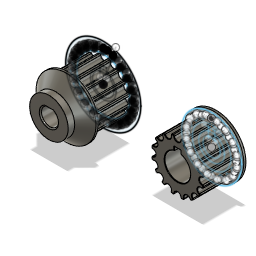
htd5m (Autodesk Fusion 360 design; units mm, degrees)
Autodesk Fusion 360 part; units mm, degrees
sketch "Sketch1" plane through (0, 0, 0) normal (0, 0, 1) x (1, 0, 0)
  circle A0 centre (0, 0) radius 15.345 construction
  circle A1 centre (0, 0) radius 13.285 construction
  line L0 (0, 0) -> (0, 15.345) construction
  circle A2 centre (0, 14.81) radius 1.525 construction
  line L1 (0, 0) -> (5.8121, 17.8879)
  circle A3 centre (4.5765, 14.0851) radius 1.525 construction
  circle A4 centre (2.7586, 14.6956) radius 0.3927 construction
  circle A5 centre (1.9549, 14.7863) radius 0.43 construction
  arc A6 (0, 13.285) -> (1.5249, 14.7915) centre (0, 14.81) ccw
  arc A7 (2.0112, 15.2126) -> (1.5249, 14.7915) centre (1.9549, 14.7863) ccw
  arc A8 (3.1309, 14.5706) -> (2.8311, 15.0816) centre (2.7586, 14.6956) ccw
  arc A9 (3.1309, 14.5706) -> (4.1053, 12.6348) centre (4.5765, 14.0851) ccw
  line L2 (2.8311, 15.0816) -> (2.0112, 15.2126)
  arc A10 (-1.5249, 14.825) -> (0, 13.285) centre (0, 14.81) ccw
  arc A11 (-1.5249, 14.825) -> (-1.968, 15.2183) centre (-1.9176, 14.8288) ccw
  line L3 (-1.968, 15.2183) -> (-2.7882, 15.0896)
  arc A12 (-2.7882, 15.0896) -> (-3.1206, 14.5388) centre (-2.7101, 14.6667) ccw
  arc A13 (-4.1053, 12.6348) -> (-3.1206, 14.5388) centre (-4.5765, 14.0851) ccw
  arc A14 (-6.0315, 13.6282) -> (-4.1053, 12.6348) centre (-4.5765, 14.0851) ccw
  arc A15 (-6.0315, 13.6282) -> (-6.5743, 13.8653) centre (-6.4061, 13.5105) ccw
  line L4 (-6.5743, 13.8653) -> (-7.3147, 13.4894)
  arc A16 (-7.3147, 13.4894) -> (-7.4606, 12.8629) centre (-7.1097, 13.1114) ccw
  arc A17 (-7.8087, 10.7478) -> (-7.4606, 12.8629) centre (-8.7051, 11.9815) ccw
  arc A18 (-9.9476, 11.0973) -> (-7.8087, 10.7478) centre (-8.7051, 11.9815) ccw
  arc A19 (-9.9476, 11.0973) -> (-10.5372, 11.1551) centre (-10.2675, 10.8697) ccw
  line L5 (-10.5372, 11.1551) -> (-11.1251, 10.5689)
  arc A20 (-11.1251, 10.5689) -> (-11.0703, 9.9279) centre (-10.8134, 10.2727) ccw
  arc A21 (-10.7478, 7.8087) -> (-11.0703, 9.9279) centre (-11.9815, 8.7051) ccw
  arc A22 (-12.89, 7.4802) -> (-10.7478, 7.8087) centre (-11.9815, 8.7051) ccw
  arc A23 (-12.89, 7.4802) -> (-13.4686, 7.353) centre (-13.1239, 7.1648) ccw
  line L6 (-13.4686, 7.353) -> (-13.8466, 6.6137)
  arc A24 (-13.8466, 6.6137) -> (-13.5964, 6.0211) centre (-13.4586, 6.4284) ccw
  arc A25 (-12.6348, 4.1053) -> (-13.5964, 6.0211) centre (-14.0851, 4.5765) ccw
  arc A26 (-14.5706, 3.1309) -> (-12.6348, 4.1053) centre (-14.0851, 4.5765) ccw
  arc A27 (-14.5706, 3.1309) -> (-15.0816, 2.8311) centre (-14.6956, 2.7586) ccw
  line L7 (-15.0816, 2.8311) -> (-15.2126, 2.0112)
  arc A28 (-15.2126, 2.0112) -> (-14.7915, 1.5249) centre (-14.7863, 1.9549) ccw
  arc A29 (-13.285, 0) -> (-14.7915, 1.5249) centre (-14.81, 0) ccw
  arc A30 (-14.825, -1.5249) -> (-13.285, 0) centre (-14.81, 0) ccw
  arc A31 (-14.825, -1.5249) -> (-15.2183, -1.968) centre (-14.8288, -1.9176) ccw
  line L8 (-15.2183, -1.968) -> (-15.0896, -2.7882)
  arc A32 (-15.0896, -2.7882) -> (-14.5388, -3.1206) centre (-14.6667, -2.7101) ccw
  arc A33 (-12.6348, -4.1053) -> (-14.5388, -3.1206) centre (-14.0851, -4.5765) ccw
  arc A34 (-13.6282, -6.0315) -> (-12.6348, -4.1053) centre (-14.0851, -4.5765) ccw
  arc A35 (-13.6282, -6.0315) -> (-13.8653, -6.5743) centre (-13.5105, -6.4061) ccw
  line L9 (-13.8653, -6.5743) -> (-13.4894, -7.3147)
  arc A36 (-13.4894, -7.3147) -> (-12.8629, -7.4606) centre (-13.1114, -7.1097) ccw
  arc A37 (-10.7478, -7.8087) -> (-12.8629, -7.4606) centre (-11.9815, -8.7051) ccw
  arc A38 (-11.0973, -9.9476) -> (-10.7478, -7.8087) centre (-11.9815, -8.7051) ccw
  arc A39 (-11.0973, -9.9476) -> (-11.1551, -10.5372) centre (-10.8697, -10.2675) ccw
  line L10 (-11.1551, -10.5372) -> (-10.5689, -11.1251)
  arc A40 (-10.5689, -11.1251) -> (-9.9279, -11.0703) centre (-10.2727, -10.8134) ccw
  arc A41 (-7.8087, -10.7478) -> (-9.9279, -11.0703) centre (-8.7051, -11.9815) ccw
  arc A42 (-7.4802, -12.89) -> (-7.8087, -10.7478) centre (-8.7051, -11.9815) ccw
  arc A43 (-7.4802, -12.89) -> (-7.353, -13.4686) centre (-7.1648, -13.1239) ccw
  line L11 (-7.353, -13.4686) -> (-6.6137, -13.8466)
  arc A44 (-6.6137, -13.8466) -> (-6.0211, -13.5964) centre (-6.4284, -13.4586) ccw
  arc A45 (-4.1053, -12.6348) -> (-6.0211, -13.5964) centre (-4.5765, -14.0851) ccw
  arc A46 (-3.1309, -14.5706) -> (-4.1053, -12.6348) centre (-4.5765, -14.0851) ccw
  arc A47 (-3.1309, -14.5706) -> (-2.8311, -15.0816) centre (-2.7586, -14.6956) ccw
  line L12 (-2.8311, -15.0816) -> (-2.0112, -15.2126)
  arc A48 (-2.0112, -15.2126) -> (-1.5249, -14.7915) centre (-1.9549, -14.7863) ccw
  arc A49 (0, -13.285) -> (-1.5249, -14.7915) centre (0, -14.81) ccw
  arc A50 (1.5249, -14.825) -> (0, -13.285) centre (0, -14.81) ccw
  arc A51 (1.5249, -14.825) -> (1.968, -15.2183) centre (1.9176, -14.8288) ccw
  line L13 (1.968, -15.2183) -> (2.7882, -15.0896)
  arc A52 (2.7882, -15.0896) -> (3.1206, -14.5388) centre (2.7101, -14.6667) ccw
  arc A53 (4.1053, -12.6348) -> (3.1206, -14.5388) centre (4.5765, -14.0851) ccw
  arc A54 (6.0315, -13.6282) -> (4.1053, -12.6348) centre (4.5765, -14.0851) ccw
  arc A55 (6.0315, -13.6282) -> (6.5743, -13.8653) centre (6.4061, -13.5105) ccw
  line L14 (6.5743, -13.8653) -> (7.3147, -13.4894)
  arc A56 (7.3147, -13.4894) -> (7.4606, -12.8629) centre (7.1097, -13.1114) ccw
  arc A57 (7.8087, -10.7478) -> (7.4606, -12.8629) centre (8.7051, -11.9815) ccw
  arc A58 (9.9476, -11.0973) -> (7.8087, -10.7478) centre (8.7051, -11.9815) ccw
  arc A59 (9.9476, -11.0973) -> (10.5372, -11.1551) centre (10.2675, -10.8697) ccw
  line L15 (10.5372, -11.1551) -> (11.1251, -10.5689)
  arc A60 (11.1251, -10.5689) -> (11.0703, -9.9279) centre (10.8134, -10.2727) ccw
  arc A61 (10.7478, -7.8087) -> (11.0703, -9.9279) centre (11.9815, -8.7051) ccw
  arc A62 (12.89, -7.4802) -> (10.7478, -7.8087) centre (11.9815, -8.7051) ccw
  arc A63 (12.89, -7.4802) -> (13.4686, -7.353) centre (13.1239, -7.1648) ccw
  line L16 (13.4686, -7.353) -> (13.8466, -6.6137)
  arc A64 (13.8466, -6.6137) -> (13.5964, -6.0211) centre (13.4586, -6.4284) ccw
  arc A65 (12.6348, -4.1053) -> (13.5964, -6.0211) centre (14.0851, -4.5765) ccw
  arc A66 (14.5706, -3.1309) -> (12.6348, -4.1053) centre (14.0851, -4.5765) ccw
  arc A67 (14.5706, -3.1309) -> (15.0816, -2.8311) centre (14.6956, -2.7586) ccw
  line L17 (15.0816, -2.8311) -> (15.2126, -2.0112)
  arc A68 (15.2126, -2.0112) -> (14.7915, -1.5249) centre (14.7863, -1.9549) ccw
  arc A69 (13.285, 0) -> (14.7915, -1.5249) centre (14.81, 0) ccw
  arc A70 (14.825, 1.5249) -> (13.285, 0) centre (14.81, 0) ccw
  arc A71 (14.825, 1.5249) -> (15.2183, 1.968) centre (14.8288, 1.9176) ccw
  line L18 (15.2183, 1.968) -> (15.0896, 2.7882)
  arc A72 (15.0896, 2.7882) -> (14.5388, 3.1206) centre (14.6667, 2.7101) ccw
  arc A73 (12.6348, 4.1053) -> (14.5388, 3.1206) centre (14.0851, 4.5765) ccw
  arc A74 (13.6282, 6.0315) -> (12.6348, 4.1053) centre (14.0851, 4.5765) ccw
  arc A75 (13.6282, 6.0315) -> (13.8653, 6.5743) centre (13.5105, 6.4061) ccw
  line L19 (13.8653, 6.5743) -> (13.4894, 7.3147)
  arc A76 (13.4894, 7.3147) -> (12.8629, 7.4606) centre (13.1114, 7.1097) ccw
  arc A77 (10.7478, 7.8087) -> (12.8629, 7.4606) centre (11.9815, 8.7051) ccw
  arc A78 (11.0973, 9.9476) -> (10.7478, 7.8087) centre (11.9815, 8.7051) ccw
  arc A79 (11.0973, 9.9476) -> (11.1551, 10.5372) centre (10.8697, 10.2675) ccw
  line L20 (11.1551, 10.5372) -> (10.5689, 11.1251)
  arc A80 (10.5689, 11.1251) -> (9.9279, 11.0703) centre (10.2727, 10.8134) ccw
  arc A81 (7.8087, 10.7478) -> (9.9279, 11.0703) centre (8.7051, 11.9815) ccw
  arc A82 (7.4802, 12.89) -> (7.8087, 10.7478) centre (8.7051, 11.9815) ccw
  arc A83 (7.4802, 12.89) -> (7.353, 13.4686) centre (7.1648, 13.1239) ccw
  line L21 (7.353, 13.4686) -> (6.6137, 13.8466)
  arc A84 (6.6137, 13.8466) -> (6.0211, 13.5964) centre (6.4284, 13.4586) ccw
  arc A85 (4.1053, 12.6348) -> (6.0211, 13.5964) centre (4.5765, 14.0851) ccw
  circle A86 centre (0, 0) radius 17.5
  circle A87 centre (0, 0) radius 5
  line L22 (2.1794, 4.5) -> (-2.1794, 4.5)
  circle A88 centre (0, 0) radius 6
  line L23 (-1.5, 7.48) -> (1.5, 7.48)
  line L24 (-1.5, 7.48) -> (-1.5, 2.3316)
  line L25 (1.5, 7.48) -> (1.5, 3.2749)
  circle A89 centre (0, 0) radius 12.3184
  circle A90 centre (50.6261, -0.0294) radius 10.15 construction
  line L26 (50.6261, -0.0294) -> (50.6261, 12.1806) construction
  arc A91 (48.6006, 12.0114) -> (49.1018, 11.6002) centre (48.672, 11.5873) ccw construction
  arc A92 (49.1018, 11.6002) -> (48.6006, 12.0114) centre (48.672, 11.5873) ccw
  arc A93 (49.1683, 12.0932) -> (48.6006, 12.0114) centre (50.6261, -0.0294) ccw
  arc A94 (52.6516, 12.0114) -> (52.1504, 11.6002) centre (52.5802, 11.5873) ccw
  arc A95 (52.1504, 11.6002) -> (52.6516, 12.0114) centre (52.5802, 11.5873) ccw construction
  arc A96 (48.6006, 12.0114) -> (52.6516, 12.0114) centre (50.6261, -0.0294) ccw
  arc A97 (52.0839, 12.0932) -> (49.1683, 12.0932) centre (50.6261, -0.0294) ccw
  arc A98 (52.6516, 12.0114) -> (52.0839, 12.0932) centre (50.6261, -0.0294) ccw
  arc A99 (52.0839, 12.0932) -> (49.1683, 12.0932) centre (50.6261, 11.6456) ccw construction
  arc A100 (49.1683, 12.0932) -> (49.1018, 11.6002) centre (50.6261, 11.6456) ccw
  arc A101 (52.1504, 11.6002) -> (52.0839, 12.0932) centre (50.6261, 11.6456) ccw
  arc A102 (50.6261, 10.1206) -> (52.1504, 11.6002) centre (50.6261, 11.6456) ccw
  arc A103 (49.1018, 11.6002) -> (50.6261, 10.1206) centre (50.6261, 11.6456) ccw
  arc A104 (44.7674, 10.1316) -> (46.7419, 9.3479) centre (46.1583, 10.7569) ccw
  arc A105 (46.7419, 9.3479) -> (47.5839, 11.2982) centre (46.1583, 10.7569) ccw
  arc A106 (47.8896, 11.8699) -> (47.5839, 11.2982) centre (47.9859, 11.4509) ccw
  arc A107 (44.7674, 10.1316) -> (44.147, 10.3197) centre (44.3752, 9.9553) ccw
  arc A108 (41.3249, 7.1161) -> (43.449, 7.1477) centre (42.3706, 8.226) ccw
  arc A109 (43.449, 7.1477) -> (43.4806, 9.2718) centre (42.3706, 8.226) ccw
  arc A110 (43.5442, 9.9169) -> (43.4806, 9.2718) centre (43.7936, 9.5667) ccw
  arc A111 (41.3249, 7.1161) -> (40.6797, 7.0525) centre (41.03, 6.8031) ccw
  arc A112 (39.2984, 3.0127) -> (41.2487, 3.8548) centre (39.8398, 4.4384) ccw
  arc A113 (41.2487, 3.8548) -> (40.4651, 5.8293) centre (39.8398, 4.4384) ccw
  arc A114 (40.2769, 6.4497) -> (40.4651, 5.8293) centre (40.6414, 6.2215) ccw
  arc A115 (39.2984, 3.0127) -> (38.7267, 2.7071) centre (39.1458, 2.6107) ccw
  arc A116 (38.9965, -1.5538) -> (40.4761, -0.0294) centre (38.9511, -0.0294) ccw
  arc A117 (40.4761, -0.0294) -> (38.9965, 1.4949) centre (38.9511, -0.0294) ccw
  arc A118 (38.5853, 1.996) -> (38.9965, 1.4949) centre (39.0093, 1.9247) ccw
  arc A119 (38.9965, -1.5538) -> (38.5853, -2.0549) centre (39.0093, -1.9836) ccw
  arc A120 (40.4651, -5.8882) -> (41.2487, -3.9137) centre (39.8398, -4.4973) ccw
  arc A121 (41.2487, -3.9137) -> (39.2984, -3.0716) centre (39.8398, -4.4973) ccw
  arc A122 (38.7267, -2.766) -> (39.2984, -3.0716) centre (39.1458, -2.6696) ccw
  arc A123 (40.4651, -5.8882) -> (40.2769, -6.5085) centre (40.6414, -6.2804) ccw
  arc A124 (43.4806, -9.3307) -> (43.449, -7.2066) centre (42.3706, -8.2849) ccw
  arc A125 (43.449, -7.2066) -> (41.3249, -7.1749) centre (42.3706, -8.2849) ccw
  arc A126 (40.6797, -7.1114) -> (41.3249, -7.1749) centre (41.03, -6.862) ccw
  arc A127 (43.4806, -9.3307) -> (43.5442, -9.9758) centre (43.7936, -9.6255) ccw
  arc A128 (47.5839, -11.3571) -> (46.7419, -9.4068) centre (46.1583, -10.8157) ccw
  arc A129 (46.7419, -9.4068) -> (44.7674, -10.1904) centre (46.1583, -10.8157) ccw
  arc A130 (44.147, -10.3786) -> (44.7674, -10.1904) centre (44.3752, -10.0141) ccw
  arc A131 (47.5839, -11.3571) -> (47.8896, -11.9288) centre (47.9859, -11.5098) ccw
  arc A132 (52.1504, -11.659) -> (50.6261, -10.1794) centre (50.6261, -11.7044) ccw
  arc A133 (50.6261, -10.1794) -> (49.1018, -11.659) centre (50.6261, -11.7044) ccw
  arc A134 (48.6006, -12.0703) -> (49.1018, -11.659) centre (48.672, -11.6462) ccw
  arc A135 (52.1504, -11.659) -> (52.6516, -12.0703) centre (52.5802, -11.6462) ccw
  arc A136 (56.4849, -10.1904) -> (54.5103, -9.4068) centre (55.0939, -10.8157) ccw
  arc A137 (54.5103, -9.4068) -> (53.6683, -11.3571) centre (55.0939, -10.8157) ccw
  arc A138 (53.3627, -11.9288) -> (53.6683, -11.3571) centre (53.2663, -11.5098) ccw
  arc A139 (56.4849, -10.1904) -> (57.1052, -10.3786) centre (56.877, -10.0141) ccw
  arc A140 (59.9273, -7.1749) -> (57.8032, -7.2066) centre (58.8816, -8.2849) ccw
  arc A141 (57.8032, -7.2066) -> (57.7716, -9.3307) centre (58.8816, -8.2849) ccw
  arc A142 (57.708, -9.9758) -> (57.7716, -9.3307) centre (57.4586, -9.6255) ccw
  arc A143 (59.9273, -7.1749) -> (60.5725, -7.1114) centre (60.2222, -6.862) ccw
  arc A144 (61.9538, -3.0716) -> (60.0035, -3.9137) centre (61.4124, -4.4973) ccw
  arc A145 (60.0035, -3.9137) -> (60.7871, -5.8882) centre (61.4124, -4.4973) ccw
  arc A146 (60.9753, -6.5085) -> (60.7871, -5.8882) centre (60.6108, -6.2804) ccw
  arc A147 (61.9538, -3.0716) -> (62.5255, -2.766) centre (62.1064, -2.6696) ccw
  arc A148 (62.2557, 1.4949) -> (60.7761, -0.0294) centre (62.3011, -0.0294) ccw
  arc A149 (60.7761, -0.0294) -> (62.2557, -1.5538) centre (62.3011, -0.0294) ccw
  arc A150 (62.6669, -2.0549) -> (62.2557, -1.5538) centre (62.2429, -1.9836) ccw
  arc A151 (62.2557, 1.4949) -> (62.6669, 1.996) centre (62.2429, 1.9247) ccw
  arc A152 (60.7871, 5.8293) -> (60.0035, 3.8548) centre (61.4124, 4.4384) ccw
  arc A153 (60.0035, 3.8548) -> (61.9538, 3.0127) centre (61.4124, 4.4384) ccw
  arc A154 (62.5255, 2.7071) -> (61.9538, 3.0127) centre (62.1064, 2.6107) ccw
  arc A155 (60.7871, 5.8293) -> (60.9753, 6.4497) centre (60.6108, 6.2215) ccw
  arc A156 (57.7716, 9.2718) -> (57.8032, 7.1477) centre (58.8816, 8.226) ccw
  arc A157 (57.8032, 7.1477) -> (59.9273, 7.1161) centre (58.8816, 8.226) ccw
  arc A158 (60.5725, 7.0525) -> (59.9273, 7.1161) centre (60.2222, 6.8031) ccw
  arc A159 (57.7716, 9.2718) -> (57.708, 9.9169) centre (57.4586, 9.5667) ccw
  arc A160 (53.6683, 11.2982) -> (54.5103, 9.3479) centre (55.0939, 10.7569) ccw
  arc A161 (54.5103, 9.3479) -> (56.4849, 10.1316) centre (55.0939, 10.7569) ccw
  arc A162 (57.1052, 10.3197) -> (56.4849, 10.1316) centre (56.877, 9.9553) ccw
  arc A163 (53.6683, 11.2982) -> (53.3627, 11.8699) centre (53.2663, 11.4509) ccw
  circle A164 centre (50.6261, -0.0294) radius 4
  circle A165 centre (50.6261, -0.0294) radius 6
  line L27 (48.6896, 3.4706) -> (52.5626, 3.4706)
  line L28 (47.069, 7.4506) -> (54.0561, 7.4506)
  line L29 (49.1261, 7.4506) -> (49.1261, 2.8308)
  line L30 (52.1261, 7.4506) -> (52.1261, 2.9509)
  circle A166 centre (50.6261, -0.0294) radius 14
  circle A167 centre (50.6261, -0.0294) radius 9
  dimension "d1" = 30.69
  dimension "d3" = 3.05
  dimension "d6" = 26.57
  dimension "d7" = 18
  dimension "d8" = 3.05
  dimension "d9" = 0.86
  dimension "d11" = 360
  dimension "d14" = 35
  dimension "d17" = 10
  dimension "d18" = 4.5
  dimension "d22" = 12
  dimension "d23" = 1.5
  dimension "d24" = 1.5
  dimension "d25" = 7.48
  dimension "d44" = 24.42
  dimension "d45" = 20.3
  dimension "d46" = 3.05
  dimension "d47" = 0.86
  dimension "d48" = 0.86
  dimension "d50" = 360
  dimension "d51" = 8
  dimension "d52" = 12
  dimension "d53" = 3.5
  dimension "d54" = 7.48
  dimension "d55" = 1.5
  dimension "d56" = 1.5
  dimension "d57" = 28
  dimension "d74" = 18
  constraint coincident A0.centre A1.centre
  constraint coincident A0 L0.end
  constraint vertical L0
  constraint coincident L0 A2.centre
  constraint tangent A1 A2
  constraint coincident L1 A3.centre
  constraint tangent A1 A3
  constraint tangent A3 A4
  constraint tangent A0 A4
  constraint tangent A0 A5
  constraint tangent A2 A5
  constraint coincident A2 A6.end
  constraint coincident A5 A6.end
  constraint coincident A1 A6.start
  constraint coincident L0 A6.start
  constraint coincident A5.centre A7.centre
  constraint coincident A0 A8.end
  constraint coincident A4 A8.end
  constraint coincident A4.centre A8.centre
  constraint coincident A3 A9.end
  constraint coincident A1 A9.end
  constraint coincident L1 A9.end
  constraint coincident A3.centre A9.centre
  constraint concentric A0 A86
  constraint concentric A86 A87
  constraint coincident A87 L22.start
  constraint coincident A87 L22.end
  constraint horizontal L22
  constraint concentric A86 A88
  constraint perpendicular L0 L23
  constraint perpendicular L23 L24
  constraint perpendicular L23 L25
  constraint concentric A86 A89
  constraint concentric A90 A96
  constraint coincident A90.centre L26.start
  constraint coincident L26.end A96
  constraint vertical L26
  constraint coincident L26 A99.centre
  constraint tangent A90 A100
  constraint tangent A94 A96
  constraint tangent A94 A100
  constraint tangent A91 A96
  constraint tangent A91 A100
  constraint concentric A91 A92
  constraint concentric A93 A96
  constraint coincident A94.end A100
  constraint concentric A94 A95
  constraint concentric A96 A97
  constraint concentric A96 A98
  constraint concentric A99 A100
  constraint coincident A90 A102.start
  constraint concentric A100 A101
  constraint concentric A100 A102
  constraint concentric A100 A103
  constraint concentric A98 A164
  constraint concentric A98 A165
  constraint coincident A164 L27.start
  constraint coincident A164 L27.end
  constraint horizontal L27
  constraint perpendicular L26 L28
  constraint coincident L28 L29.start
  constraint perpendicular L28 L29
  constraint coincident L28 L30.start
  constraint perpendicular L28 L30
  constraint concentric A165 A166
  constraint concentric A90 A167
  measures "d1" diameter of A0
  measures "d3" diameter of A2
  measures "d6" diameter of A1
  measures "d7" angle of L0 L1
  measures "d8" diameter of A3
  measures "d9" diameter of A5
  measures "d14" diameter of A86
  measures "d17" diameter of A87
  measures "d18" distance of A0.centre L22
  measures "d22" diameter of A88
  measures "d23" distance of L0 L24
  measures "d24" distance of L0 L25
  measures "d25" distance of A0.centre L23
  measures "d44" diameter of A96
  measures "d45" diameter of A90
  measures "d46" diameter of A100
  measures "d47" diameter of A94
  measures "d48" diameter of A91
  measures "d51" diameter of A164
  measures "d52" diameter of A165
  measures "d53" distance of A90.centre L27
  measures "d54" distance of A90.centre L28
  measures "d55" distance of L26 L30
  measures "d56" distance of L26 L29
  measures "d57" diameter of A166
  measures "d74" diameter of A167
extrude "Extrude7" add sketch "Sketch1" along normal blind 16 contours A92 A94 A96 A102 A103 A104 A105 A106 A107 A108 A109 A110 A111 A112 A113 A114 A115 A116 A117 A118 A119 A120 A121 A122 A123 A124 A125 A126 A127 A128 A129 A130 A131 A132 A133 A134 A135 A136 A137 A138 A139 A140 A141 A142 A143 A144 A145 A146 A147 A148 A149 A150 A151 A152 A153 A154 A155 A156 A157 A158 A159 A160 A161 A162 A163 | A167 makes body 1
extrude "Extrude2" add sketch "Sketch1" against normal blind 2 separate body contours L1 A87 L22 L24 L25 | L1 L22 L25 | A87 L22 | L1 A87 L25 | L1 A87 L22 L25 | A87 L22 L24 | L1 A87 A88 L25 | L1 A87 A88 L24 | A87 A88 L24 L25 | A88 L23 L24 L25 | A6 A7 A8 A9 L2 A10 A11 L3 A12 A13 A14 A15 L4 A16 A17 A18 A19 L5 A20 A21 A22 A23 L6 A24 A25 A26 A27 L7 A28 A29 A30 A31 L8 A32 A33 A34 A35 L9 A36 A37 A38 A39 L10 A40 A41 A42 A43 L11 A44 A45 A46 A47 L12 A48 A49 A50 A51 L13 A52 A53 A54 A55 L14 A56 A57 A58 A59 L15 A60 A61 A62 A63 L16 A64 A65 A66 A67 L17 A68 A69 A70 A71 L18 A72 A73 A74 A75 L19 A76 A77 A78 A79 L20 A80 A81 A82 A83 L21 A84 A85 | A86 | A89 makes body 2
extrude "Extrude1" add sketch "Sketch1" along normal blind 16 separate body contours L1 A87 L22 L24 L25 | L1 L22 L25 | A87 L22 | L1 A87 L25 | L1 A87 L22 L25 | A87 L22 L24 | L1 A87 A88 L25 | L1 A87 A88 L24 | A87 A88 L24 L25 | A88 L23 L24 L25 | A6 A7 A8 A9 L2 A10 A11 L3 A12 A13 A14 A15 L4 A16 A17 A18 A19 L5 A20 A21 A22 A23 L6 A24 A25 A26 A27 L7 A28 A29 A30 A31 L8 A32 A33 A34 A35 L9 A36 A37 A38 A39 L10 A40 A41 A42 A43 L11 A44 A45 A46 A47 L12 A48 A49 A50 A51 L13 A52 A53 A54 A55 L14 A56 A57 A58 A59 L15 A60 A61 A62 A63 L16 A64 A65 A66 A67 L17 A68 A69 A70 A71 L18 A72 A73 A74 A75 L19 A76 A77 A78 A79 L20 A80 A81 A82 A83 L21 A84 A85 | A89 makes body 3
extrude "Extrude3" cut sketch "Sketch1" along normal blind 120 from surface at -2 contours A87 L22 bodies 2 3
combine "Combine1" operation add target body 3 tool bodies 2
extrude "Extrude4" add sketch "Sketch1" along normal blind 16 from surface at 80 separate body contours A6 A7 A8 A9 L2 A10 A11 L3 A12 A13 A14 A15 L4 A16 A17 A18 A19 L5 A20 A21 A22 A23 L6 A24 A25 A26 A27 L7 A28 A29 A30 A31 L8 A32 A33 A34 A35 L9 A36 A37 A38 A39 L10 A40 A41 A42 A43 L11 A44 A45 A46 A47 L12 A48 A49 A50 A51 L13 A52 A53 A54 A55 L14 A56 A57 A58 A59 L15 A60 A61 A62 A63 L16 A64 A65 A66 A67 L17 A68 A69 A70 A71 L18 A72 A73 A74 A75 L19 A76 A77 A78 A79 L20 A80 A81 A82 A83 L21 A84 A85 | A89 makes body 4
extrude "Extrude5" add sketch "Sketch1" against normal blind 2 from surface at 80 contours A6 A7 A8 A9 L2 A10 A11 L3 A12 A13 A14 A15 L4 A16 A17 A18 A19 L5 A20 A21 A22 A23 L6 A24 A25 A26 A27 L7 A28 A29 A30 A31 L8 A32 A33 A34 A35 L9 A36 A37 A38 A39 L10 A40 A41 A42 A43 L11 A44 A45 A46 A47 L12 A48 A49 A50 A51 L13 A52 A53 A54 A55 L14 A56 A57 A58 A59 L15 A60 A61 A62 A63 L16 A64 A65 A66 A67 L17 A68 A69 A70 A71 L18 A72 A73 A74 A75 L19 A76 A77 A78 A79 L20 A80 A81 A82 A83 L21 A84 A85 | A86 | A89 bodies 4
extrude "Extrude6" add sketch "Sketch1" against normal blind 8 from surface at -2 contours L1 A87 L22 L24 L25 | L1 L22 L25 | L1 A87 L25 | L1 A87 L22 L25 | A87 L22 L24 | L1 A87 A88 L25 | L1 A87 A88 L24 | A87 A88 L24 L25 | A88 L23 L24 L25 | A89 bodies 3
chamfer "Chamfer1" distance 5 angle 45 1 edges at (-11.4848, -4.4545, -2) on bodies 3
fillet "Fillet1" radius 1 1 edges at (-16.3157, 6.3283, -2) on bodies 3
fillet "Fillet2" radius 1 1 edges at (-11.4848, -4.4545, -7) on bodies 3
fillet "Fillet3" radius 1 1 edges at (-16.3157, -6.3283, 0) on bodies 3
fillet "Fillet4" radius 0.3 1 faces at (0.0324, 7.4294, 16) on bodies 3
extrude "Extrude8" add sketch "Sketch1" against normal blind 2 contours A92 A94 A96 A102 A103 A104 A105 A106 A107 A108 A109 A110 A111 A112 A113 A114 A115 A116 A117 A118 A119 A120 A121 A122 A123 A124 A125 A126 A127 A128 A129 A130 A131 A132 A133 A134 A135 A136 A137 A138 A139 A140 A141 A142 A143 A144 A145 A146 A147 A148 A149 A150 A151 A152 A153 A154 A155 A156 A157 A158 A159 A160 A161 A162 A163 | A92 A93 A100 | A97 A100 A101 A102 A103 | A96 A104 A105 A106 A107 | A94 A98 A101 | A96 A108 A109 A110 A111 | A96 A160 A161 A162 A163 | A96 A112 A113 A114 A115 | A96 A156 A157 A158 A159 | A96 A116 A117 A118 A119 | A96 A152 A153 A154 A155 | A96 A120 A121 A122 A123 | A96 A148 A149 A150 A151 | A96 A124 A125 A126 A127 | A96 A144 A145 A146 A147 | A96 A128 A129 A130 A131 | A96 A140 A141 A142 A143 | A96 A132 A133 A134 A135 | A96 A136 A137 A138 A139 | A166 | A167 bodies 1
fillet "Fillet5" radius 0.2 1 faces at (43.3178, 4.8257, 16) on bodies 1
fillet "Fillet6" radius 1 1 edges at (37.5735, -5.0921, 0) on bodies 1
fillet "Fillet7" radius 0.5 4 edges at (50.6261, -6.0294, -2) (49.1261, 6.6153, -2) (50.6261, 7.4506, -2) (52.1261, 6.6153, -2) on bodies 1
extrude "Extrude9" add sketch "Sketch1" against normal blind 16 from surface at -20 separate body contours A92 A94 A96 A102 A103 A104 A105 A106 A107 A108 A109 A110 A111 A112 A113 A114 A115 A116 A117 A118 A119 A120 A121 A122 A123 A124 A125 A126 A127 A128 A129 A130 A131 A132 A133 A134 A135 A136 A137 A138 A139 A140 A141 A142 A143 A144 A145 A146 A147 A148 A149 A150 A151 A152 A153 A154 A155 A156 A157 A158 A159 A160 A161 A162 A163 | A164 A165 L29 L30 | A164 L27 L30 | A164 L27 L29 | A164 L27 L29 L30 | A164 A165 L29 L30 | A165 L28 L29 L30 | A167 makes body 5
extrude "Extrude10" add sketch "Sketch1" along normal blind 2 from surface at -20 contours A92 A94 A96 A102 A103 A104 A105 A106 A107 A108 A109 A110 A111 A112 A113 A114 A115 A116 A117 A118 A119 A120 A121 A122 A123 A124 A125 A126 A127 A128 A129 A130 A131 A132 A133 A134 A135 A136 A137 A138 A139 A140 A141 A142 A143 A144 A145 A146 A147 A148 A149 A150 A151 A152 A153 A154 A155 A156 A157 A158 A159 A160 A161 A162 A163 | A92 A93 A100 | A97 A100 A101 A102 A103 | A96 A104 A105 A106 A107 | A94 A98 A101 | A96 A108 A109 A110 A111 | A96 A160 A161 A162 A163 | A96 A112 A113 A114 A115 | A96 A156 A157 A158 A159 | A96 A116 A117 A118 A119 | A96 A152 A153 A154 A155 | A96 A120 A121 A122 A123 | A96 A148 A149 A150 A151 | A96 A124 A125 A126 A127 | A96 A144 A145 A146 A147 | A96 A128 A129 A130 A131 | A96 A140 A141 A142 A143 | A96 A132 A133 A134 A135 | A96 A136 A137 A138 A139 | A164 A165 L29 L30 | A164 L27 L30 | A164 L27 L29 | A164 L27 L29 L30 | A164 A165 L29 L30 | A165 L28 L29 L30 | A166 | A167 bodies 5
extrude "Extrude11" add sketch "Sketch1" along normal blind 8 from surface at -18 contours A164 A165 L29 L30 | A164 L27 L30 | A164 L27 L29 | A164 L27 L29 L30 | A164 A165 L29 L30 | A165 L28 L29 L30 | A167 bodies 5
chamfer "Chamfer2" distance 5 angle 45 1 edges at (42.2352, 3.2251, -18) on bodies 5
fillet "Fillet8" radius 0.5 2 edges at (50.6261, -4.0294, -10) (50.6261, 3.4706, -10) on bodies 5
fillet "Fillet9" radius 1 1 edges at (37.5735, 5.0332, -20) on bodies 5
fillet "Fillet10" radius 0.3 1 faces at (50.6634, 5.6886, -36) on bodies 5
move_body "Move1" bodies 5 to x (1, 0, 0) y (0, 1, 0) z (0, 0, 1) at (-50, 0, 36)
hidden bodies 3 4
equation "d6 = 30.69 mm - ( 2.06 * 2 ) * 1 mm"
equation "d7 = ( 360 / 20 ) * 1 deg"
equation "d25 = 13.48 mm - 6 mm"
equation "d44 = ( 12.21 * 2 ) * 1 mm"
equation "d45 = 24.42 mm - ( 2.06 * 2 ) * 1 mm"
